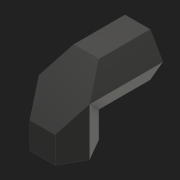
# Autodesk Inventor part: link_a0
Saved by Autodesk Inventor 2017 (Build 210142000, 142)
## iProperties
Created: 2019-08-03
Part Number: link_a0
Material: ABS Plastic
Document SubType Name: Modeling
Designer: Dell
Density: 1.06 g/cm^3
Appearance: Smooth - Black
Author: Dell
Autodesk Inventor part; units mm, degrees
ref_plane "YZ Plane" through (0, 0, 0) normal (1, 0, 0) x (0, 1, 0)
ref_plane "XZ Plane" through (0, 0, 0) normal (0, 1, 0) x (-1, 0, 0)
ref_plane "XY Plane" through (0, 0, 0) normal (0, 0, 1) x (1, 0, 0)
sketch "Sketch1" plane through (0, 0, 0) normal (0, 0, 1) x (1, 0, 0)
  line L0 (57.5, 0) -> (28.75, -49.7965)
  line L1 (28.75, -49.7965) -> (-28.75, -49.7965)
  line L2 (-28.75, -49.7965) -> (-57.5, 0)
  line L3 (-57.5, 0) -> (-28.75, 49.7965)
  line L4 (-28.75, 49.7965) -> (28.75, 49.7965)
  line L5 (28.75, 49.7965) -> (57.5, 0)
  point P0 (0, 0)
  point P1 (0, 0)
  dimension "d0" = 115
  constraints: 12 end point, 1 coincident, 13 other
  measures "d0" distance of L0.start L2.end
extrude "Extrusion1" add sketch "Sketch1" along normal blind 159.4929
sketch "Sketch2" plane through (-28.75, -49.7965, 0) normal (0, -1, 0) x (1, 0, 0)
  line L0 (-28.75, 109.6965) -> (0, 159.4929)
  line L1 (0, 159.4929) -> (57.5, 159.4929)
  line L2 (57.5, 159.4929) -> (86.25, 109.6965)
  line L3 (86.25, 109.6965) -> (57.5, 59.9)
  line L4 (57.5, 59.9) -> (0, 59.9)
  line L5 (0, 59.9) -> (-28.75, 109.6965)
  line L6 (0, 159.4929) -> (57.5, 159.4929) projected
  point P0 (28.75, 0)
  point P1 (28.75, 109.6965)
  point P2 (28.75, 159.4929)
  dimension "d3" = 115
  constraints: 12 end point, 2 midpoint, 1 point on line, 13 other
  measures "d3" distance of L2.end L0.start
extrude "Extrusion2" add sketch "Sketch2" against normal blind 216.6673
sketch "Sketch9" plane through (0, 0, 0) normal (1, 0, 0) x (0, 1, 0)
  line L0 (0, 109.6965) -> (-49.7965, 59.9) projected
  line L1 (-49.7965, 109.6965) -> (0, 109.6965) projected
  line L2 (-49.7965, 59.9) -> (-49.7965, 109.6965) projected
  line L3 (-49.7965, 159.4929) -> (0, 109.6965) projected
  line L4 (-49.7965, 109.6965) -> (-49.7965, 159.4929) projected
  line L5 (-49.7965, 109.6965) -> (0, 109.6965) projected
  line L6 (-49.7965, 159.4929) -> (0, 109.6965) projected
  line L7 (0, 109.6965) -> (0, 159.4929) projected
  line L8 (-49.7965, 159.4929) -> (0, 159.4929) projected
  line L9 (0, 109.6965) -> (49.7965, 159.4929) projected
  line L10 (0, 159.4929) -> (49.7965, 159.4929) projected
  line L11 (0, 109.6965) -> (0, 159.4929) projected
  point P0 (0, 0)
extrude "Extrusion8" cut sketch "Sketch9" along normal through all both and the other way through all
body "Solid1"
